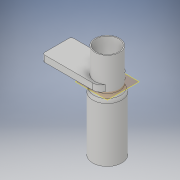
# Autodesk Inventor part: Elbow Extension
Saved by Autodesk Inventor 2019 (Build 230136000, 136)
## iProperties
Created: 2020-04-29
Part Number: Elbow Extension
Material: Generic
Document SubType Name: Modeling
Designer: Kepler
Density: 1 g/cm^3
Appearance: Default
Author: Kepler
Autodesk Inventor part; units mm, degrees
ref_plane "YZ Plane" through (0, 0, 0) normal (1, 0, 0) x (0, 1, 0)
ref_plane "XY Plane" through (0, 0, 0) normal (0, 0, 1) x (1, 0, 0)
sketch "Sketch1" plane through (0, 0, 0) normal (0, 1, 0) x (-1, 0, 0)
  circle A0 centre (0, 0) radius 10
  circle A1 centre (0, 0) radius 11.5
  dimension "d0" = 20
  dimension "d1" = 23
  constraints: 2 centre point, 2 coincident
  measures "d0" diameter of A0
  measures "d1" diameter of A1
extrude "Extrusion1" add sketch "Sketch1" along normal blind 40
sketch "Sketch2" plane through (0, 40, 0) normal (0, 1, 0) x (1, 0, 0)
  circle A0 centre (0, 0) radius 9.75
  circle A1 centre (0, 0) radius 9
  dimension "d4" = 19.5
  constraints: 2 centre point, 2 coincident
  measures "d4" diameter of A0
extrude "Extrusion2" add sketch "Sketch2" along normal blind 35
sketch "Sketch3" plane through (0, 40, 0) normal (0, 1, 0) x (1, 0, 0)
  circle A0 centre (0, 0) radius 9.75 projected
  circle A1 centre (0, 0) radius 11.5 projected
extrude "Extrusion3" add sketch "Sketch3" along normal blind 5
fillet "Fillet1" radius 5 2 edges at (-9.75, 45, 0) (-11.5, 45, 0)
fillet "Fillet2" radius 5 2 edges at (-9, 40, 0) (10, 40, 0)
ref_plane "Work Plane1" through (0, 50, 0) normal (0, 1, 0) x (-1, 0, 0)
sketch "Sketch4" plane through (0, 50, 0) normal (0, 1, 0) x (-1, 0, 0)
  circle A0 centre (0, 0) radius 11.5 projected
  line L0 (0, -11.5) -> (38, -11.5)
  line L1 (40, -9.5) -> (40, 9.5)
  line L2 (38, 11.5) -> (0, 11.5)
  arc A1 (40, 9.5) -> (38, 11.5) centre (38, 9.5) ccw
  arc A2 (38, -11.5) -> (40, -9.5) centre (38, -9.5) ccw
  circle A3 centre (0, 0) radius 9.75 projected
  spline S0 degree 2 poles (0, -11.5) (-3.8325, -11.5) (-6, -7.6852) knots 0 0 0 1 1 1
  spline S1 degree 2 poles (0, 11.5) (-3.8325, 11.5) (-6, 7.6852) knots 0 0 0 1 1 1
  point P0 (40, -11.5)
  dimension "d19" = 40
  dimension "d20" = 2
  constraints: 6 end point, 6 point on circle, 5 horizontal, 4 tangent, 2 centre point, 2 perpendicular, 2 point on line, 1 equal radius, 1 vertical alignment, 5 other
  measures "d19" distance of L0.start point (40, -11.5)
  measures "d20" radius of A1
extrude "Extrusion5" add sketch "Sketch4" along normal blind 5 contours A0 S0 A3 S1 | A0 L2 A1 L1 A2 L0 picked at (10.8206, -0.853)
body "Solid1"
